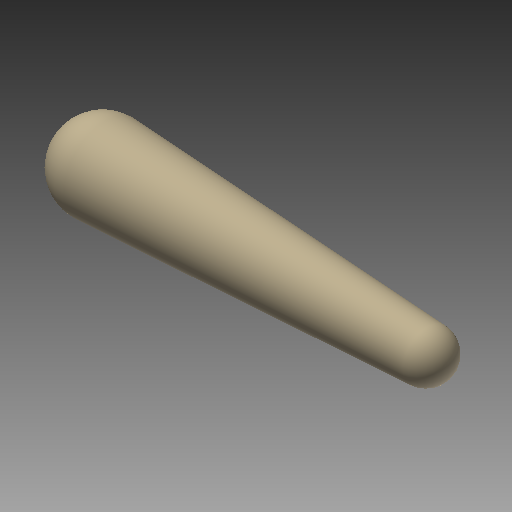
# Autodesk Inventor part: 3D HUMAN
Saved by Autodesk Inventor 2019 (Build 230136000, 136)
## iProperties
Category: PART
Shininess: 64.0
Length Units: 11272
Angle Units: 11279
Time Units: 11290
Mass Units: 11286
Length Display Precision: 3
Angle Display Precision: 2
Compacted: True
Part Number: 3D HUMAN
Document SubType Name: Modeling
Created: 2003-03-23
Designer: M.F.
Catalog Web Link: www.apollocanard.com
Density: 1 g/cm^3
Material: Generic
Appearance: Beige
Density: 0.0
Volumn: 0.0
Area: 0.0
PropertySet Name: Model Information
Control State: 0
Master: False
Checked Out: False
Title: iMan
Author: M.F.
Autodesk Inventor part; units mm, degrees
ref_plane "YZ Plane" through (0, 0, 0) normal (1, 0, 0) x (0, 1, 0)
ref_plane "XZ Plane" through (0, 0, 0) normal (0, 1, 0) x (-1, 0, 0)
ref_plane "XY Plane" through (0, 0, 0) normal (0, 0, 1) x (1, 0, 0)
sketch "Sketch1" plane through (0, 0, 0) normal (0, 0, 1) x (1, 0, 0)
  circle A0 centre (0, 0) radius 61.468
  circle A1 centre (0, -482.6) radius 36.576
  line L0 (0, 61.468) -> (0, -519.176)
  line L1 (61.3862, -3.1705) -> (36.5273, -484.4866)
  dimension "d17" = 122.936
  dimension "d18" = 73.152
  dimension "d20" = 519.176
  constraints: 4 end point, 4 point on circle, 2 centre point, 2 tangent, 1 coincident, 1 point on line, 1 vertical, 1 vertical alignment
  measures "d17" diameter of A0
  measures "d18" diameter of A1
  measures "d20" distance of L0.end A0.centre
revolve "Revolution1" add sketch "Sketch1" angle 360 about axis through (0, 61.468, 0) along (0, -1, 0) picked at (13.1703, 15.6957) picked at (21.0091, -490.665) contours A0 L0 | L1 A1 L0 A0 | A1 L0
equation "\"d17\" = KNEE_THK"
equation "\"d18\" = ANKLE_THK"
equation "\"d20\" = KNEE_TO_FOOT"
equation "\"d16\" = ELBOW_TO_WRIST"
equation "\"KNEE_THK\" = 122.936"
equation "\"ANKLE_THK\" = 73.152"
equation "\"KNEE_TO_FOOT\" = 519.176"
equation "\"ELBOW_TO_WRIST\" = 260.096"
body "Solid1"
